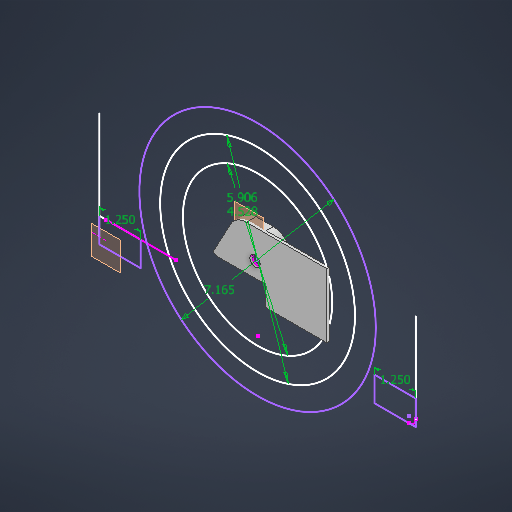
# Autodesk Inventor part: MISLcase
Saved by Autodesk Inventor 2026.1 (Build 301233020, 233B)
## iProperties
Created: 2026-09-24
Part Number: MISLcase
Material: Generic
Document SubType Name: Modeling
Density: 1 g/cm^3
Appearance: Default
Autodesk Inventor part; units mm, degrees
ref_plane "YZ Plane" through (0, 0, 0) normal (1, 0, 0) x (0, 1, 0)
ref_plane "XZ Plane" through (0, 0, 0) normal (0, 1, 0) x (-1, 0, 0)
ref_plane "XY Plane" through (0, 0, 0) normal (0, 0, 1) x (1, 0, 0)
ref_plane "Work Plane1" through (-116.713, 0, 25.019) normal (0, 0, 1) x (1, 0, 0)
sketch "Sketch1" plane through (-116.713, 0, 25.019) normal (0, 0, 1) x (1, 0, 0)
  circle A0 centre (116.713, 50.8) radius 4.826 projected
  circle A1 centre (116.713, 50.8) radius 91
  line L0 (-5.08, 5.08) -> (-5.08, 87.3153)
  arc A2 (233.426, 0) -> (238.506, 5.08) centre (233.426, 5.08) ccw projected
  line L1 (238.506, 5.08) -> (238.506, 73.9139)
  line L2 (53.9374, 19.05) -> (0, 19.05) projected
  line L3 (-5.08, 0) -> (26.67, 0)
  line L4 (26.67, 0) -> (26.67, 19.05)
  line L5 (26.67, 19.05) -> (-5.08, 19.05)
  line L6 (-5.08, 19.05) -> (-5.08, 0)
  line L7 (238.506, 0) -> (206.756, 0)
  line L8 (206.756, 0) -> (206.756, 19.05)
  line L9 (206.756, 19.05) -> (238.506, 19.05)
  line L10 (238.506, 19.05) -> (238.506, 0)
  circle A3 centre (116.713, 50.8) radius 3.9687 projected
  circle A4 centre (116.713, 50.8) radius 75
  circle A5 centre (116.713, 50.8) radius 57.5
  point P0 (116.713, 0)
  point P1 (233.426, 0)
  point P2 (-5.08, 19.05)
  dimension "d1" = 182
  dimension "d2" = 31.75
  dimension "d3" = 31.75
  dimension "d20" = 150
  dimension "d21" = 115
  constraints: 20 end point, 4 parallel, 3 centre point, 3 coincident, 2 horizontal, 2 perpendicular, 2 vertical, 1 point on circle, 1 point on line, 1 tangent
  measures "d1" diameter of A1
  measures "d2" distance of L5.end L4.end
  measures "d3" distance of L8.end L9.end
  measures "d20" diameter of A4
  measures "d21" diameter of A5
ref_plane "Work Plane6" through (-6.6254, 69.85, 25.019) normal (0, 0, 1) x (1, 0, 0)
ref_plane "Work Plane4" through (-6.6254, 69.85, 25.019) normal (0, 0, 1) x (1, 0, 0)
sketch "Sketch6" plane through (-6.6254, 69.85, 25.019) normal (0, 0, 1) x (1, 0, 0)
  line L0 (-22.5883, -30.7335) -> (-8.9499, -5.3511) projected
  arc A0 (0, 0) -> (-8.9499, -5.3511) centre (0, -10.16) ccw projected
  arc A1 (22.2006, -5.3511) -> (13.2508, 0) centre (13.2508, -10.16) ccw projected
  line L1 (0, 0) -> (13.2508, 0) projected
  line L2 (22.2006, -5.3511) -> (35.8391, -30.7335) projected
  arc A2 (35.8391, -30.7335) -> (69.401, -50.8) centre (69.401, -12.7) ccw projected
  arc A3 (-56.1502, -50.8) -> (-22.5883, -30.7335) centre (-56.1502, -12.7) ccw projected
  arc A4 (36.2795, -30.4968) -> (69.401, -50.3) centre (69.401, -12.7) ccw
  line L3 (36.2795, -30.4968) -> (22.6411, -5.1144)
  arc A5 (22.6411, -5.1144) -> (13.2508, 0.5) centre (13.2508, -10.16) ccw
  line L4 (13.2508, 0.5) -> (0, 0.5)
  arc A6 (0, 0.5) -> (-9.3903, -5.1144) centre (0, -10.16) ccw
  line L5 (-9.3903, -5.1144) -> (-23.0287, -30.4968)
  arc A7 (-56.1502, -50.3) -> (-23.0287, -30.4968) centre (-56.1502, -12.7) ccw
  arc A8 (-56.1502, -47.3) -> (-25.6714, -29.0769) centre (-56.1502, -12.7) ccw
  line L6 (-25.6714, -29.0769) -> (-12.033, -3.6945)
  arc A9 (0, 3.5) -> (-12.033, -3.6945) centre (0, -10.16) ccw
  line L7 (0, 3.5) -> (13.2508, 3.5)
  arc A10 (25.2837, -3.6945) -> (13.2508, 3.5) centre (13.2508, -10.16) ccw
  line L8 (25.2837, -3.6945) -> (38.9222, -29.0769)
  arc A11 (38.9222, -29.0769) -> (69.401, -47.3) centre (69.401, -12.7) ccw
  line L9 (-25.6714, -29.0769) -> (-23.0287, -30.4968)
  line L10 (49.4158, -40.9445) -> (47.986, -43.6056)
  point P0 (6.6254, -69.85)
  dimension "d22" = 0.5
  dimension "d23" = 3
  constraints: 18 point on circle, 16 end point, 8 centre point, 12 other
  measures "d22" distance between parallel lines of L1 L4
  measures "d23" distance between parallel lines of L5 L6
extrude "Extrusion5" add sketch "Sketch6" against normal blind 5.5
ref_plane "Work Plane7" through (-6.6254, 69.85, 25.019) normal (0, 0, 1) x (1, 0, 0)
sketch "Sketch7" plane through (-6.6254, 69.85, 25.019) normal (0, 0, 1) x (1, 0, 0)
  line L0 (-25.6714, -29.0769) -> (-23.0287, -30.4968) projected
  line L1 (-23.0287, -30.4968) -> (14.4045, -30.4968)
  line L2 (14.4045, -30.4968) -> (14.4045, 0.4374)
  arc A0 (22.6411, -5.1144) -> (13.2508, 0.5) centre (13.2508, -10.16) ccw projected
  line L3 (14.4045, -30.4968) -> (14.4045, -45.9071)
  line L4 (14.4045, -45.9071) -> (62.0107, -45.9071)
  line L5 (13.2508, 3.5) -> (0, 3.5) projected
  line L6 (0, 3.5) -> (62.0107, 3.5)
  line L7 (62.0107, 3.5) -> (62.0107, -45.9071)
  circle A1 centre (6.6254, -19.05) radius 3.9687 projected
  line L8 (-23.0287, -30.4968) -> (-25.6714, -29.0769)
  line L9 (-12.033, -3.6945) -> (-25.6714, -29.0769) projected
  arc A2 (0, 3.5) -> (-12.033, -3.6945) centre (0, -10.16) ccw projected
  point P0 (6.6254, -69.85)
  constraints: 14 end point, 3 perpendicular, 2 horizontal, 1 collinear, 1 point on circle, 1 vertical
extrude "Extrusion6" add sketch "Sketch7" along normal blind 2
body "Solid1"
